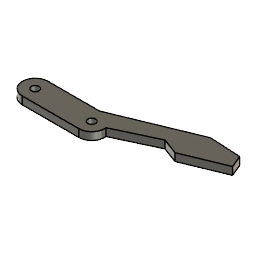
GripperP1 (Autodesk Fusion 360 design; units mm, degrees)
part number: 2026-06-13-12-36-49-281
Autodesk Fusion 360 part; units mm, degrees
sketch "Sketch1" plane through (0, 0, 0) normal (0, 0, 1) x (1, 0, 0)
  line L0 (0, -5) -> (22, -5)
  arc A0 (22, -5) -> (22, 5) centre (22, 0) ccw
  line L1 (22, 5) -> (0, 5)
  arc A1 (0, 5) -> (0, -5) centre (0, 0) ccw
  line L2 (0, 0) -> (22, 0) construction
  circle A2 centre (0, 0) radius 1.5
  line L3 (20.05, 5) -> (60.7446, 21.7316)
  line L4 (60.7446, 21.7316) -> (64.6864, 12.1444)
  line L5 (64.6864, 12.1444) -> (23.9013, -4.6244)
  line L6 (50.6615, 17.5859) -> (62.7155, 16.938)
  line L7 (48.8067, 5.6155) -> (42.5976, 7.9233)
  line L8 (42.5976, 7.9233) -> (26.963, 0.6072)
  circle A3 centre (22, 0) radius 1.5
  dimension "d1" = 22
  dimension "d2" = 5
  dimension "d3" = 3
  dimension "d4" = 157.65
  dimension "d5" = 44
  dimension "d6" = 1.95
  dimension "d7" = 3
  constraint tangent L0 A0
  constraint tangent A0 L1
  constraint parallel L0 L1
  constraint tangent L1 A1
  constraint tangent L0 A1
  constraint horizontal L2
  constraint coincident A1.centre L2.start
  constraint concentric A1 A2
  constraint coincident L1 L3.start
  constraint coincident A0 L5.end
  constraint perpendicular L3 L4
  constraint perpendicular L4 L5
  constraint tangent A0 L5
  constraint coincident L3 L6.start
  constraint midpoint L4 L6.end
  constraint coincident L5 L7.start
  constraint coincident A0 L8.end
  constraint concentric A0 A3
  measures "d1" distance of A1.centre A0.centre
  measures "d2" radius of A1
  measures "d3" diameter of A2
  measures "d4" angle of L1 L3
  measures "d5" distance of L3.start L3.end
  measures "d6" horizontal distance of A0.centre L3.start
  measures "d7" diameter of A3
extrude "Extrude1" add sketch "Sketch1" along normal blind 3 contours L0 A0 L1 A1 | A0 L1 L3 L4 L5 L6 L7 L8
sketch "Sketch2" plane through (0, 0, 0) normal (0, 0, 1) x (1, 0, 0)
  circle A0 centre (14, 12) radius 3.5
  circle A1 centre (14, 12) radius 1.5
  circle A2 centre (45, 12) radius 1.5
  circle A3 centre (45, 12) radius 3.5
  line L0 (14, 12) -> (45, 12)
  line L1 (17.1623, 13.5) -> (41.8377, 13.5)
  line L2 (17.1623, 10.5) -> (41.8377, 10.5)
  dimension "d10" = 3
  dimension "d11" = 3
  dimension "d12" = 7
  dimension "d13" = 7
  dimension "d14" = 31
  dimension "d15" = 1.5
  constraint concentric A0 A1
  constraint concentric A2 A3
  constraint coincident A0.centre A1.centre
  constraint coincident A2.centre A3.centre
  constraint horizontal L0
  constraint coincident A0 L1.start
  constraint coincident A3 L1.end
  constraint horizontal L1
  constraint symmetric L0 L1.start L2.start
  constraint symmetric L0 L1.end L2.end
  measures "d10" diameter of A1
  measures "d11" diameter of A2
  measures "d12" diameter of A0
  measures "d13" diameter of A3
  measures "d14" distance of A0.centre A2.centre
  measures "d15" distance of L0 L1
